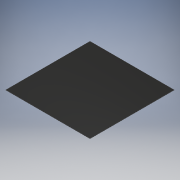
# Autodesk Inventor part: Cover
Saved by Autodesk Inventor 2019.3 (Build 233278000, 278)
## iProperties
Created: 2019-01-14
Part Number: Cover
Material: ABS-Kunststoff
Document SubType Name: Modeling
Designer: Jonas
Density: 1.06 g/cm^3
Appearance: Glänzend - Schwarz
Author: Jonas
Autodesk Inventor part; units mm, degrees
ref_plane "YZ Plane" through (0, 0, 0) normal (1, 0, 0) x (0, 1, 0)
ref_plane "XZ Plane" through (0, 0, 0) normal (0, 1, 0) x (-1, 0, 0)
ref_plane "XY Plane" through (0, 0, 0) normal (0, 0, 1) x (1, 0, 0)
sketch "Skizze1" plane through (0, 0, 0) normal (0, 1, 0) x (-1, 0, 0)
  line L0 (71.3648, 125.2628) -> (-192.6352, 125.2628)
  line L1 (-192.6352, 125.2628) -> (-192.6352, -138.7372)
  line L2 (-192.6352, -138.7372) -> (71.3648, -138.7372)
  line L3 (71.3648, -138.7372) -> (71.3648, 125.2628)
  point P0 (0, 0)
  dimension "d0" = 264
  dimension "d1" = 264
  constraints: 8 end point, 2 parallel, 1 horizontal, 1 perpendicular
  measures "d0" distance of L2.end L0.start
  measures "d1" distance of L1.end L2.end
extrude "Extrusion1" add sketch "Skizze1" along normal blind 1
